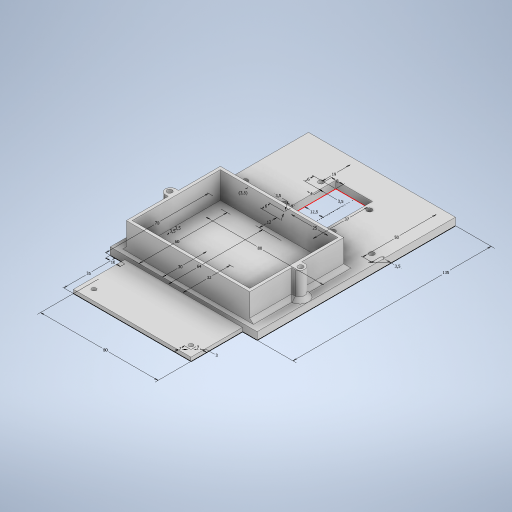
# Autodesk Inventor part: peca_principal
Saved by Autodesk Inventor 2024.3 (Build 283343000, 343)
## iProperties
Created: 2024-11-18
Part Number: peca_principal
Material: Genérico
Document SubType Name: Modeling
Designer: lostv
Density: 1 g/cm^3
Appearance: Padrão
Author: lostv
Autodesk Inventor part; units mm, degrees
ref_plane "YZ Plane" through (0, 0, 0) normal (1, 0, 0) x (0, 1, 0)
ref_plane "XZ Plane" through (0, 0, 0) normal (0, 1, 0) x (-1, 0, 0)
ref_plane "XY Plane" through (0, 0, 0) normal (0, 0, 1) x (1, 0, 0)
sketch "Esboço1" plane through (0, 0, 0) normal (0, 1, 0) x (-1, 0, 0)
  line L0 (0, 0) -> (80, 0)
  line L1 (80, -170) -> (0, -170)
  line L2 (80, -40) -> (0, -40)
  line L3 (0, -40) -> (0, -100)
  line L4 (0, -100) -> (80, -100)
  line L5 (80, -100) -> (80, -40)
  line L6 (80, 0) -> (80, -35)
  line L7 (80, -35) -> (90, -35)
  line L8 (90, -35) -> (90, -105)
  line L9 (80, 0) -> (80, -35)
  line L10 (80, -40) -> (80, -100)
  line L11 (90, -70) -> (0, -70)
  line L12 (40, 0) -> (40, -170)
  line L13 (0, -35) -> (-10, -35)
  line L14 (-10, -35) -> (-10, -105)
  line L15 (0, -35) -> (0, 0)
  line L16 (0, -100) -> (0, -40)
  line L17 (52.5, -114) -> (27.5, -114)
  line L18 (27.5, -114) -> (27.5, -151)
  line L19 (27.5, -151) -> (52.5, -151)
  line L20 (52.5, -151) -> (52.5, -114)
  line L21 (82, -38) -> (-2, -38)
  line L22 (-2, -102) -> (82, -102)
  circle A0 centre (84.5595, -70) radius 1.75
  line L23 (84.5595, -66.5) -> (82, -66.5)
  line L24 (82, -73.5) -> (84.5595, -73.5)
  arc A1 (84.5595, -73.5) -> (84.5595, -66.5) centre (83.9005, -70) ccw
  line L25 (82, -102) -> (82, -73.5)
  line L26 (82, -66.5) -> (82, -38)
  circle A2 centre (-4.5595, -70) radius 1.75
  line L27 (-4.5595, -66.5) -> (-2, -66.5)
  line L28 (-2, -73.5) -> (-4.5595, -73.5)
  arc A3 (-4.5595, -66.5) -> (-4.5595, -73.5) centre (-3.9005, -70) ccw
  line L29 (-2, -38) -> (-2, -66.5)
  line L30 (-2, -73.5) -> (-2, -102)
  line L31 (90, -105) -> (90, -151)
  line L32 (90, -151) -> (90, -170)
  line L33 (90, -170) -> (-10, -170)
  line L34 (-10, -170) -> (-10, -105)
  line L35 (80, -35) -> (0, -35)
  circle A4 centre (-3, -120) radius 1.75
  circle A5 centre (83, -120) radius 1.75
  circle A6 centre (7, -7) radius 1.5
  circle A7 centre (73, -7) radius 1.5
  line L36 (52.5, -114) -> (60.5, -114)
  line L37 (60.5, -114) -> (60.5, -151)
  line L38 (60.5, -151) -> (52.5, -151)
  line L39 (52.5, -151) -> (52.5, -114)
  circle A8 centre (56.5, -120) radius 1.75
  circle A9 centre (56.5, -145) radius 1.75
  line L40 (27.5, -114) -> (19.5, -114)
  line L41 (19.5, -114) -> (19.5, -151)
  line L42 (19.5, -151) -> (27.5, -151)
  circle A10 centre (23.5, -120) radius 1.75
  circle A11 centre (23.5, -145) radius 1.75
  point P0 (45, -70)
  point P1 (40, -102)
  point P2 (80, -17.5)
  point P3 (0, -170)
  point P4 (56.5, -114)
  point P5 (56.5, -151)
  dimension "d3" = 60
  dimension "d4" = 35
  dimension "d5" = 10
  dimension "d6" = 70
  dimension "d7" = 30
  dimension "d9" = 80
  dimension "d12" = 64
  dimension "d13" = 32
  dimension "d15" = 3.5
  dimension "d16" = 3.5
  dimension "d17" = 37
  dimension "d18" = 25
  dimension "d19" = 12.5
  dimension "d21" = 19
  dimension "d22" = 12
  dimension "d23" = 80
  dimension "d30" = 3.5
  dimension "d31" = 7
  dimension "d32" = 50
  dimension "d33" = 3
  dimension "d35" = 3.5
  dimension "d36" = 7
  dimension "d37" = 7
  dimension "d54" = 8
  dimension "d55" = 3.5
  dimension "d56" = 3.5
  dimension "d57" = 6
  dimension "d58" = 6
  dimension "d59" = 4
  dimension "d60" = 4
  dimension "d63" = 135
  constraints: 86 end point, 18 parallel, 16 symmetric about line, 12 centre point, 12 perpendicular, 9 midpoint, 8 horizontal, 4 point on circle, 2 collinear, 2 point on line, 1 vertical, 6 other
  measures "d3" distance of L4.end L2.start
  measures "d4" distance of L6.end L0.end
  measures "d5" distance of L6.end L7.end
  measures "d6" distance of L7.end L8.end
  measures "d7" distance between parallel lines of L2 L11
  measures "d9" distance between parallel lines of L3 L10
  measures "d12" distance between parallel lines of L22 L21
  measures "d13" distance from line of point (45, -70) L21
  measures "d15" distance from line of A0.centre L23
  measures "d16" distance from line of A0.centre L24
  measures "d17" distance between parallel lines of L19 L17
  measures "d18" distance between parallel lines of L18 L20
  measures "d19" distance between parallel lines of L20 L12
  measures "d21" distance between parallel lines of L1 L19
  measures "d22" distance from line of L17 point (40, -102)
  measures "d23" distance from line of L15 point (80, -17.5)
  measures "d30" diameter of A4
  measures "d31" distance from line of A4.centre L34
  measures "d32" distance from line of L33 A4.centre
  measures "d33" diameter of A6
  measures "d35" diameter of A5
  measures "d36" distance from line of L15 A6.centre
  measures "d37" distance from line of L0 A6.centre
  measures "d54" distance of L37.end L38.end
  measures "d55" diameter of A8
  measures "d56" diameter of A9
  measures "d57" distance of point (56.5, -114) A8.centre
  measures "d58" distance of point (56.5, -151) A9.centre
  measures "d59" distance from line of L37 A9.centre
  measures "d60" distance from line of L37 A8.centre
  measures "d63" distance between parallel lines of L33 L13
extrude "Extrusão1" add sketch "Esboço1" along normal blind 23 contours L21 L26 L23 A1 L11 A0 L5 L2 L12 | L12 L2 L3 L4 L22 L30 L28 A3 L27 L29 L21 | A1 L24 L25 L22 L12 L4 L5 L11 A0
extrude "Extrusão4" add sketch "Esboço1" along normal blind 2.5 contours L0 L12 L35 L15 | L0 L6 L35 L12
extrude "Extrusão5" add sketch "Esboço1" along normal blind 5 contours L35 L12 L21 L29 L27 A3 L28 L30 L22 L17 L40 L41 L42 L19 L1 L33 L34 L14 L13 | L35 L7 L8 L11 A1 L23 L26 L21 L12 | L12 L11 L3 L2 | L2 L5 L11 L12 | L8 L31 L32 L33 L1 L12 L19 L38 L37 L36 L17 L22 L25 L24 A1 L11 | L12 L4 L3 L11 | L11 L5 L4 L12 | L42 L41 L40 L18 | L20 L36 L37 L38 | A8 | A9 | A10 | A11
chamfer "Chanfro1" distance 2.5 angle 45 1 edges at (-40, 5, -102)
chamfer "Chanfro2" distance 2.5 angle 45 5 edges at (2, 5, -103.25) (2, 5, -87.75) (7.462, 5, -70) (3.2797, 5, -73.5) (2, 5, -52.25)
chamfer "Chanfro3" distance 2.5 angle 45 2 edges at (4.5297, 5, -66.5) (6.7045, 5, -66.5)
chamfer "Chanfro4" distance 2.5 angle 45 6 edges at (-82, 5, -87.75) (-82, 5, -103.25) (-87.462, 5, -70) (-82, 5, -52.25) (-83.2797, 5, -73.5) (-83.2797, 5, -66.5)
extrude "Extrusão6" cut sketch "Esboço1" along normal mid plane 10 contours A8 | A9 | A10 | A11
